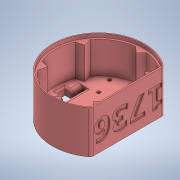
# Autodesk Inventor part: camHolderBottom
Saved by Autodesk Inventor 2020 (Build 240168000, 168)
## iProperties
Created: 2020-02-08
Part Number: camHolderBottom
Material: Generic
Document SubType Name: Modeling
Designer: Chris Gerth
Density: 1 g/cm^3
Appearance: Default(1)
Author: Chris Gerth
Autodesk Inventor part; units mm, degrees
ref_plane "YZ Plane" through (0, 0, 0) normal (1, 0, 0) x (0, 1, 0)
ref_plane "XZ Plane" through (0, 0, 0) normal (0, 1, 0) x (-1, 0, 0)
ref_plane "XY Plane" through (0, 0, 0) normal (0, 0, 1) x (1, 0, 0)
sketch "Sketch1" plane through (0, 0, 0) normal (0, 1, 0) x (-1, 0, 0)
  arc A0 (-25.4, -31.7246) -> (-25.4, 31.7246) centre (0, 0) ccw
  line L0 (-25.4, 31.7246) -> (-25.4, -31.7246)
  dimension "d0" = 81.28
  dimension "d31" = 25.4
  constraints: 2 end point, 2 point on circle, 1 centre point, 1 coincident, 1 vertical
  measures "d0" diameter of A0
  measures "d31" distance from line of L0 point (0, 0)
extrude "Extrusion1" add sketch "Sketch1" along normal blind 6.35
sketch "Sketch2" plane through (0, 6.35, 0) normal (0, 1, 0) x (0, 0, 1)
  arc A0 (-31.7246, 25.4) -> (31.7246, 25.4) centre (0, 0) ccw
  arc A1 (-30.9461, 22.225) -> (30.9461, 22.225) centre (0, 0) ccw
  arc A2 (-31.7246, 25.4) -> (31.7246, 25.4) centre (0, 0) ccw projected
  line L0 (31.7246, 25.4) -> (-31.7246, 25.4)
  line L1 (30.9461, 22.225) -> (-30.9461, 22.225)
  dimension "d3" = 76.2
  dimension "d32" = 3.175
  constraints: 4 end point, 4 point on circle, 2 centre point, 2 coincident, 2 horizontal
  measures "d3" diameter of A1
  measures "d32" distance between parallel lines of L0 L1
extrude "Extrusion2" add sketch "Sketch2" along normal blind 27.94
sketch "Sketch3" plane through (0, 34.29, 0) normal (0, 1, 0) x (0, 0, 1)
  arc A0 (-31.7246, 25.4) -> (31.7246, 25.4) centre (0, 0) ccw
  arc A1 (-31.7246, 25.4) -> (31.7246, 25.4) centre (0, 0) ccw
  arc A2 (-31.5893, 24.13) -> (31.5893, 24.13) centre (0, 0) ccw
  arc A3 (-31.7246, 25.4) -> (31.7246, 25.4) centre (0, 0) ccw projected
  line L0 (31.7246, 25.4) -> (-31.7246, 25.4)
  line L1 (31.5893, 24.13) -> (-31.5893, 24.13)
  dimension "d6" = 79.502
  dimension "d33" = 1.27
  constraints: 6 point on circle, 4 end point, 3 centre point, 3 coincident, 2 horizontal
  measures "d6" diameter of A2
  measures "d33" distance between parallel lines of L0 L1
extrude "Extrusion3" add sketch "Sketch3" along normal blind 3.175
sketch "Sketch4" plane through (0, 6.35, 0) normal (0, 1, 0) x (0, 0, 1)
  line L0 (-14.4, 14.4) -> (14.4, 14.4)
  line L1 (14.4, 14.4) -> (14.4, -14.4)
  line L2 (14.4, -14.4) -> (-14.4, -14.4)
  line L3 (-14.4, -14.4) -> (-14.4, 14.4)
  line L4 (-14.4, 14.4) -> (14.4, -14.4) construction
  line L5 (14.4, 14.4) -> (-14.4, -14.4) construction
  circle A0 centre (-14.4, 14.4) radius 1.55
  circle A1 centre (14.4, 14.4) radius 1.55
  circle A2 centre (-14.4, -14.4) radius 1.55
  circle A3 centre (14.4, -14.4) radius 1.55
  point P0 (0, 0)
  dimension "d9" = 28.8
  dimension "d10" = 28.8
  dimension "d11" = 3.1
  dimension "d12" = 3.1
  dimension "d13" = 3.1
  dimension "d14" = 3.1
  constraints: 12 end point, 4 centre point, 4 coincident, 2 midpoint, 2 parallel, 1 horizontal, 1 perpendicular
  measures "d9" distance of L1.end L2.end
  measures "d10" distance of L2.end L0.start
  measures "d11" diameter of A0
  measures "d12" diameter of A1
  measures "d13" diameter of A2
  measures "d14" diameter of A3
extrude "Extrusion4" cut sketch "Sketch4" against normal up to surface (6.35 mm away) contours L3 A0 L0 | L0 A0 L3 | A1 L1 L0 | L0 L1 A1 | A2 L2 L3 | L3 L2 A2 | A3 L2 L1 | L1 L2 A3
sketch "Sketch5" plane through (0, 6.35, 0) normal (0, 1, 0) x (0, 0, 1)
  line L0 (12.7, -23.7415) -> (-12.7, -23.7415)
  line L1 (-12.7, -23.7415) -> (-12.7, -26.9165)
  line L2 (-12.7, -26.9165) -> (12.7, -26.9165)
  line L3 (12.7, -26.9165) -> (12.7, -23.7415)
  line L4 (12.7, -23.7415) -> (-12.7, -26.9165) construction
  line L5 (-12.7, -23.7415) -> (12.7, -26.9165) construction
  line L6 (3.5906, -33.2771) -> (3.5906, -25.329)
  line L7 (3.5906, -25.329) -> (-3.5906, -25.329)
  line L8 (-3.5906, -25.329) -> (-3.5906, -33.2771)
  line L9 (-3.5906, -33.2771) -> (3.5906, -33.2771)
  line L10 (3.5906, -33.2771) -> (-3.5906, -25.329) construction
  line L11 (3.5906, -25.329) -> (-3.5906, -33.2771) construction
  point P0 (0, 0)
  point P1 (0, -25.329)
  point P2 (0, -29.303)
  point P3 (3.5906, -26.9165)
  point P4 (-3.5906, -26.9165)
  dimension "d17" = 25.4
  dimension "d18" = 3.175
  constraints: 24 end point, 4 midpoint, 4 parallel, 2 perpendicular, 1 vertical
  measures "d17" distance of L0.start L0.end
  measures "d18" distance of L1.end L0.end
extrude "Extrusion5" cut sketch "Sketch5" against normal up to surface (6.35 mm away)
sketch "Sketch6" plane through (0, 6.35, 0) normal (0, 1, 0) x (0, 0, 1)
  line L0 (28.575, 19.05) -> (28.575, -19.05)
  line L1 (28.575, -19.05) -> (-28.575, -19.05)
  line L2 (-28.575, -19.05) -> (-28.575, 19.05)
  line L3 (-28.575, 19.05) -> (28.575, 19.05)
  line L4 (28.575, 19.05) -> (-28.575, -19.05) construction
  line L5 (28.575, -19.05) -> (-28.575, 19.05) construction
  circle A0 centre (-28.575, -19.05) radius 1.55
  circle A1 centre (-28.575, 19.05) radius 1.55
  circle A2 centre (28.575, 19.05) radius 1.55
  circle A3 centre (28.575, -19.05) radius 1.55
  point P0 (0, 0)
  dimension "d21" = 38.1
  dimension "d22" = 57.15
  dimension "d23" = 3.1
  dimension "d24" = 3.1
  dimension "d25" = 3.1
  dimension "d26" = 3.1
  constraints: 12 end point, 4 centre point, 4 coincident, 2 parallel, 1 perpendicular
  measures "d21" distance of L1.end L2.end
  measures "d22" distance of L0.end L1.end
  measures "d23" diameter of A0
  measures "d24" diameter of A1
  measures "d25" diameter of A2
  measures "d26" diameter of A3
extrude "Extrusion6" cut sketch "Sketch6" against normal up to surface (6.35 mm away) contours L3 A2 L0 | L0 A2 L3 | A3 L1 L0 | L0 L1 A3 | A1 L2 L3 | L3 L2 A1 | A0 L2 L1 | L1 L2 A0
sketch "Sketch7" plane through (25.4, 0, 31.7246) normal (1, 0, 0) x (0, 0, -1)
  line L0 (64.016, 7.7021) -> (-12.2251, 7.7021) construction
  line L1 (-12.2251, 7.7021) -> (-12.2251, 34.1724) construction
  line L2 (-12.2251, 34.1724) -> (64.016, 34.1724) construction
  line L3 (64.016, 34.1724) -> (64.016, 7.7021) construction
  line L4 (49.939, 25.8567) -> (61.6819, 25.8567)
  line L5 (61.6819, 25.8567) -> (61.6819, 22.7589)
  line L6 (61.6819, 22.7589) -> (57.9357, 22.7589)
  line L7 (57.9357, 22.7589) -> (57.9357, 13.3502)
  line L8 (57.9357, 13.3502) -> (61.6819, 13.3502)
  line L9 (61.6819, 13.3502) -> (61.6819, 10.4541)
  spline S0 degree 2 poles (61.6819, 10.4541) (60.8606, 10.4541) (59.2324, 10.2379) (58.7426, 10.0074) knots 0 0 0 1 2 2 2
  spline S1 degree 2 poles (58.7426, 10.0074) (58.1806, 9.7192) (57.5467, 8.7539) (57.489, 8.0335) knots 0 0 0 1 2 2 2
  line L10 (57.489, 8.0335) -> (53.5987, 8.0335)
  line L11 (53.5987, 8.0335) -> (53.5987, 22.7589)
  line L12 (53.5987, 22.7589) -> (49.939, 22.7589)
  line L13 (49.939, 22.7589) -> (49.939, 25.8567)
  line L14 (33.9601, 11.6067) -> (41.5533, 25.8567)
  line L15 (41.5533, 25.8567) -> (46.5098, 25.8567)
  line L16 (46.5098, 25.8567) -> (38.5708, 11.4338)
  line L17 (38.5708, 11.4338) -> (47.0429, 11.4338)
  line L18 (47.0429, 11.4338) -> (47.0429, 8.0767)
  line L19 (47.0429, 8.0767) -> (33.9601, 8.0767)
  line L20 (33.9601, 8.0767) -> (33.9601, 11.6067)
  spline S2 degree 2 poles (18.4422, 20.4679) (18.4422, 21.7791) (19.4075, 23.926) (20.3441, 24.6752) knots 0 0 0 1 2 2 2
  spline S3 degree 2 poles (20.3441, 24.6752) (21.2806, 25.4244) (23.8309, 26.2313) (25.6608, 26.2313) knots 0 0 0 1 2 2 2
  spline S4 degree 2 poles (25.6608, 26.2313) (27.7356, 26.2313) (30.7038, 25.5397) (31.6403, 25.1074) knots 0 0 0 1 2 2 2
  line L21 (31.6403, 25.1074) -> (31.6403, 21.246)
  line L22 (31.6403, 21.246) -> (31.208, 21.246)
  spline S5 degree 2 poles (31.208, 21.246) (30.2283, 21.8655) (27.5915, 22.7877) (26.4965, 22.7877) knots 0 0 0 1 2 2 2
  spline S6 degree 2 poles (26.4965, 22.7877) (25.8481, 22.7877) (24.3352, 22.5572) (23.8165, 22.1825) knots 0 0 0 1 2 2 2
  spline S7 degree 2 poles (23.8165, 22.1825) (23.4131, 21.88) (22.9232, 21.001) (22.9232, 20.2086) knots 0 0 0 1 2 2 2
  spline S8 degree 2 poles (22.9232, 20.2086) (22.9232, 19.4161) (23.6148, 18.566) (24.1911, 18.3643) knots 0 0 0 1 2 2 2
  spline S9 degree 2 poles (24.1911, 18.3643) (24.7675, 18.1626) (26.3668, 18.1194) (26.9864, 18.1194) knots 0 0 0 1 2 2 2
  line L23 (26.9864, 18.1194) -> (27.75, 18.1194)
  line L24 (27.75, 18.1194) -> (27.75, 14.9927)
  line L25 (27.75, 14.9927) -> (27.044, 14.9927)
  spline S10 degree 2 poles (27.044, 14.9927) (26.2371, 14.9927) (24.8683, 14.8486) (24.3929, 14.6325) knots 0 0 0 1 2 2 2
  spline S11 degree 2 poles (24.3929, 14.6325) (23.9174, 14.402) (23.3843, 13.5951) (23.3843, 12.9035) knots 0 0 0 1 2 2 2
  spline S12 degree 2 poles (23.3843, 12.9035) (23.3843, 12.356) (23.8886, 11.6788) (24.2488, 11.4915) knots 0 0 0 1 2 2 2
  spline S13 degree 2 poles (24.2488, 11.4915) (24.681, 11.2754) (25.8337, 11.1313) (26.2371, 11.1313) knots 0 0 0 1 2 2 2
  spline S14 degree 2 poles (26.2371, 11.1313) (26.8855, 11.1313) (28.2543, 11.4338) (28.8883, 11.6788) knots 0 0 0 1 2 2 2
  spline S15 degree 2 poles (28.8883, 11.6788) (29.3926, 11.8661) (30.4876, 12.4713) (30.747, 12.6297) knots 0 0 0 1 2 2 2
  line L26 (30.747, 12.6297) -> (31.1216, 12.6297)
  line L27 (31.1216, 12.6297) -> (31.1216, 8.8259)
  spline S16 degree 2 poles (31.1216, 8.8259) (30.1995, 8.4369) (27.0872, 7.7021) (25.4591, 7.7021) knots 0 0 0 1 2 2 2
  spline S17 degree 2 poles (25.4591, 7.7021) (23.8742, 7.7021) (21.54, 8.2496) (20.7187, 8.7827) knots 0 0 0 1 2 2 2
  spline S18 degree 2 poles (20.7187, 8.7827) (19.811, 9.3446) (18.9032, 11.0736) (18.9032, 12.1543) knots 0 0 0 1 2 2 2
  spline S19 degree 2 poles (18.9032, 12.1543) (18.9032, 13.6816) (20.6611, 15.9581) (22.1019, 16.2895) knots 0 0 0 1 2 2 2
  line L28 (22.1019, 16.2895) -> (22.1019, 16.4624)
  spline S20 degree 2 poles (22.1019, 16.4624) (21.4679, 16.5488) (20.2576, 17.0099) (19.6813, 17.5286) knots 0 0 0 1 2 2 2
  spline S21 degree 2 poles (19.6813, 17.5286) (19.1482, 17.9897) (18.4422, 19.4593) (18.4422, 20.4679) knots 0 0 0 1 2 2 2
  spline S22 degree 2 poles (2.5209, 19.8051) (2.5209, 22.6148) (6.0797, 26.2313) (9.192, 26.2313) knots 0 0 0 1 2 2 2
  spline S23 degree 2 poles (9.192, 26.2313) (10.7481, 26.2313) (13.1831, 25.338) (14.0332, 24.4591) knots 0 0 0 1 2 2 2
  spline S24 degree 2 poles (14.0332, 24.4591) (15.0418, 23.4361) (16.1224, 20.1942) (16.1224, 17.932) knots 0 0 0 1 2 2 2
  spline S25 degree 2 poles (16.1224, 17.932) (16.1224, 15.5979) (15.1138, 11.967) (13.9756, 10.5693) knots 0 0 0 1 2 2 2
  spline S26 degree 2 poles (13.9756, 10.5693) (12.8949, 9.2438) (9.3793, 7.7453) (6.9731, 7.7453) knots 0 0 0 1 2 2 2
  spline S27 degree 2 poles (6.9731, 7.7453) (6.0942, 7.7453) (4.3363, 7.9758) (4.0193, 8.0479) knots 0 0 0 1 2 2 2
  line L29 (4.0193, 8.0479) -> (4.0193, 11.5347)
  line L30 (4.0193, 11.5347) -> (4.3363, 11.5347)
  spline S28 degree 2 poles (4.3363, 11.5347) (4.6533, 11.3762) (6.0942, 10.9872) (7.0163, 10.9872) knots 0 0 0 1 2 2 2
  spline S29 degree 2 poles (7.0163, 10.9872) (9.1055, 10.9872) (11.382, 13.1917) (11.6558, 15.2377) knots 0 0 0 1 2 2 2
  spline S30 degree 2 poles (11.6558, 15.2377) (10.7769, 14.6757) (8.9758, 14.013) (7.8376, 14.013) knots 0 0 0 1 2 2 2
  spline S31 degree 2 poles (7.8376, 14.013) (6.8722, 14.013) (5.1864, 14.5317) (4.538, 15.0215) knots 0 0 0 1 2 2 2
  spline S32 degree 2 poles (4.538, 15.0215) (3.6159, 15.7276) (2.5209, 18.0185) (2.5209, 19.8051) knots 0 0 0 1 2 2 2
  spline S33 degree 2 poles (7.7223, 22.4851) (7.3765, 22.0529) (7.0019, 21.0443) (7.0019, 20.0213) knots 0 0 0 1 2 2 2
  spline S34 degree 2 poles (7.0019, 20.0213) (7.0019, 19.1568) (7.4341, 18.0329) (7.8232, 17.7015) knots 0 0 0 1 2 2 2
  spline S35 degree 2 poles (7.8232, 17.7015) (8.2266, 17.3557) (9.2208, 17.1108) (9.7827, 17.1108) knots 0 0 0 1 2 2 2
  spline S36 degree 2 poles (9.7827, 17.1108) (10.2582, 17.1108) (11.238, 17.3557) (11.6702, 17.5286) knots 0 0 0 1 2 2 2
  spline S37 degree 2 poles (11.6702, 17.5286) (11.6702, 17.6439) (11.699, 18.1914) (11.699, 18.6092) knots 0 0 0 1 2 2 2
  spline S38 degree 2 poles (11.699, 18.6092) (11.699, 20.1509) (11.1659, 22.0096) (10.7481, 22.4851) knots 0 0 0 1 2 2 2
  spline S39 degree 2 poles (10.7481, 22.4851) (10.4455, 22.8741) (9.6386, 23.2055) (9.2064, 23.2055) knots 0 0 0 1 2 2 2
  spline S40 degree 2 poles (9.2064, 23.2055) (8.8462, 23.2055) (8.0105, 22.8453) (7.7223, 22.4851) knots 0 0 0 1 2 2 2
  point P0 (31.7246, 0)
  constraints: 2 other
extrude "Extrusion7" cut sketch "Sketch7" against normal blind 1.016
fillet "Fillet1" radius 3.175 2 edges at (25.4, 18.7325, 31.7246) (25.4, 18.7325, -31.7246)
fillet "Fillet3" radius 3.175 3 edges at (-23.7415, 6.35, 0) (-26.9165, 6.35, -8.1453) (-26.9165, 6.35, 8.1453)
fillet "Fillet4" radius 1.5875 5 edges at (-33.2771, 6.35, 0) (-27.8464, 5.4201, -3.5906) (-31.6843, 6.35, -3.5906) (-27.8464, 5.4201, 3.5906) (-31.6843, 6.35, 3.5906)
sketch "Sketch9" plane through (0, 6.35, 0) normal (0, 1, 0) x (1, 0, 0)
  circle A0 centre (0, 0) radius 38.1
  arc A1 (22.225, 30.9461) -> (22.225, -30.9461) centre (0, 0) ccw projected
  line L0 (-5.0033, 37.7701) -> (0.0033, 32.9762)
  line L1 (0.0033, 32.9762) -> (4.638, 37.8166)
  line L2 (-28.5566, 16.491) -> (-30.4312, 22.925)
  line L3 (-35.2115, 14.552) -> (-28.5566, 16.491)
  line L4 (-28.5599, -16.4852) -> (-35.0692, -14.8917)
  line L5 (-30.2082, -23.218) -> (-28.5599, -16.4852)
  line L6 (-0.0033, -32.9762) -> (-4.638, -37.8166)
  line L7 (5.0033, -37.7701) -> (-0.0033, -32.9762)
  line L8 (28.5566, -16.491) -> (30.4312, -22.925)
  line L9 (35.2115, -14.552) -> (28.5566, -16.491)
  line L10 (28.5599, 16.4852) -> (35.0692, 14.8917)
  line L11 (30.2082, 23.218) -> (28.5599, 16.4852)
  line L12 (22.225, 30.9461) -> (22.225, -30.9461)
  line L13 (22.225, -30.9461) -> (22.225, 30.9461) projected
  line L14 (22.225, 26.8313) -> (18.1598, 22.5994)
  line L15 (18.1598, 22.5994) -> (22.225, 18.6943)
  line L16 (0, 0) -> (38.1, 0)
  line L17 (22.225, -26.8313) -> (18.1598, -22.5994)
  line L18 (18.1598, -22.5994) -> (22.225, -18.6943)
  dimension "d42" = 360
  constraints: 36 end point, 3 point on circle, 3 symmetric about line, 2 perpendicular, 1 centre point, 1 coincident, 1 horizontal, 1 point on line, 1 vertical, 31 other
extrude "Extrusion8" add sketch "Sketch9" along normal up to surface (27.94 mm away) contours L15 L14 L12 | L12 L17 L18 | L1 L0 A0 | A0 L6 L7 | L2 L3 A0 | A0 L4 L5
body "Solid1"
